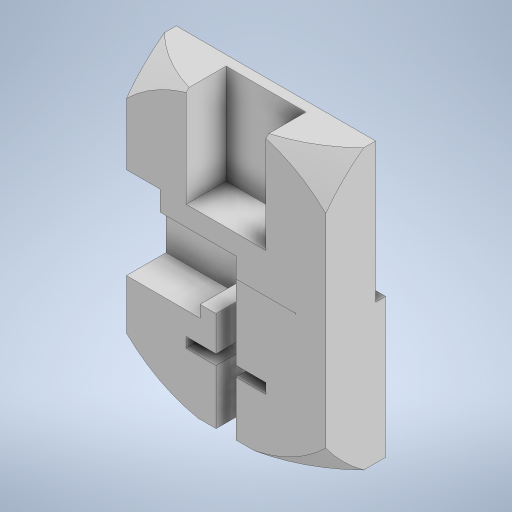
# Autodesk Inventor part: bunny head anchor
Saved by Autodesk Inventor 2024.2 (Build 282272000, 272)
## iProperties
Created: 2025-12-17
Part Number: bunny head anchor
Material: Generic
Document SubType Name: Modeling
Designer: David Toler II
Density: 1 g/cm^3
Appearance: Default
Author: David Toler II
Autodesk Inventor part; units mm, degrees
ref_plane "YZ Plane" through (0, 0, 0) normal (1, 0, 0) x (0, 1, 0)
ref_plane "XZ Plane" through (0, 0, 0) normal (0, 1, 0) x (-1, 0, 0)
ref_plane "XY Plane" through (0, 0, 0) normal (0, 0, 1) x (1, 0, 0)
sketch "Sketch1" plane through (0, 0, 0) normal (0, 0, 1) x (1, 0, 0)
  line L0 (31.75, -44.45) -> (-31.75, -44.45)
  line L1 (-31.75, -44.45) -> (-31.75, 44.45)
  line L2 (-31.75, 44.45) -> (31.75, 44.45)
  line L3 (31.75, 44.45) -> (31.75, -44.45)
  line L4 (31.75, -44.45) -> (-31.75, 44.45) construction
  line L5 (-31.75, -44.45) -> (31.75, 44.45) construction
  line L6 (-31.75, 0) -> (31.75, 0)
  line L7 (-31.75, 44.45) -> (31.75, 0)
  line L8 (-31.75, 0) -> (31.75, 44.45)
  circle A0 centre (0, 22.225) radius 11.43
  point P0 (0, 0)
  dimension "d0" = 63.5
  dimension "d1" = 44.45
  dimension "d2" = 22.86
  constraints: 18 end point, 5 midpoint, 2 parallel, 1 centre point, 1 horizontal, 1 perpendicular
  measures "d0" distance between parallel lines of L3 L1
  measures "d1" distance from line of point (0, 0) L2
  measures "d2" diameter of A0
extrude "Extrusion1" add sketch "Sketch1" along normal blind 3.175 contours L0 L1 L6 L3 | A0 L8 L7 | L7 L8 A0 | A0 L7 L8 | L8 L7 A0
sketch "Sketch2" plane through (0, 0, 3.175) normal (0, 0, 1) x (1, 0, 0)
  line L0 (31.75, -44.45) -> (31.75, 0) projected
  line L1 (31.75, 0) -> (-31.75, 0) projected
  line L2 (-31.75, 0) -> (-31.75, -44.45) projected
  line L3 (-31.75, -44.45) -> (31.75, -44.45) projected
  line L4 (-31.75, 44.45) -> (31.75, 44.45)
  line L5 (31.75, 44.45) -> (31.75, -44.45)
  line L6 (31.75, -44.45) -> (-31.75, -44.45)
  line L7 (-31.75, -44.45) -> (-31.75, 44.45)
  line L8 (-31.75, 44.45) -> (31.75, -44.45) construction
  line L9 (31.75, 44.45) -> (-31.75, -44.45) construction
  point P0 (0, 0)
  constraints: 12 end point, 2 midpoint, 2 parallel, 1 horizontal, 1 perpendicular
extrude "Extrusion2" add sketch "Sketch2" along normal blind 3.175
sketch "Sketch3" plane through (0, 0, 6.35) normal (0, 0, 1) x (1, 0, 0)
  circle A0 centre (0, -0.4493) radius 54.991
  line L0 (0, -0.4493) -> (0, 0)
  line L1 (31.75, -44.45) -> (31.75, 44.45) projected
  line L2 (31.75, 44.45) -> (-31.75, 44.45) projected
  line L3 (-31.75, 44.45) -> (-31.75, -44.45) projected
  line L4 (-31.75, -44.45) -> (31.75, -44.45) projected
  line L5 (-31.75, -44.45) -> (31.75, -44.45) projected
  line L6 (0, 44.45) -> (0, -44.45)
  line L7 (31.75, 0) -> (-31.75, 0) projected
  line L8 (-31.75, 0) -> (31.75, 0)
  line L9 (12.7, 12.7) -> (-12.7, 12.7)
  line L10 (-12.7, 12.7) -> (-12.7, 44.45)
  line L11 (-12.7, 44.45) -> (12.7, 44.45)
  line L12 (12.7, 44.45) -> (12.7, 12.7)
  line L13 (12.7, 12.7) -> (-12.7, 44.45) construction
  line L14 (-12.7, 12.7) -> (12.7, 44.45) construction
  line L15 (-33.655, 6.35) -> (-8.255, 6.35)
  line L16 (-8.255, 6.35) -> (-8.255, -16.51)
  line L17 (-8.255, -16.51) -> (-33.655, -16.51)
  line L18 (-33.655, -16.51) -> (-33.655, 6.35)
  line L19 (-8.255, 6.35) -> (31.75, 6.35)
  line L20 (-8.255, -12.7) -> (-3.175, -12.7)
  line L21 (-3.175, -12.7) -> (-3.175, -44.45)
  line L22 (-20.955, 6.35) -> (-20.955, 12.7)
  line L23 (-20.955, 12.7) -> (-31.75, 12.7)
  line L24 (3.175, 6.35) -> (3.175, -44.45)
  point P0 (0, -55.4403)
  point P1 (0, 28.575)
  point P2 (3.175, -44.45)
  point P3 (-3.175, -44.45)
  point P4 (-31.75, -16.51)
  dimension "d8" = 109.982
  dimension "d9" = 25.4
  dimension "d10" = 31.75
  dimension "d11" = 25.4
  dimension "d12" = 8.255
  dimension "d13" = 6.35
  dimension "d14" = 22.86
  dimension "d15" = 5.08
  dimension "d16" = 19.05
  dimension "d17" = 6.35
  constraints: 38 end point, 9 point on line, 6 perpendicular, 5 midpoint, 4 horizontal, 4 parallel, 2 point on circle, 2 vertical, 1 centre point
  measures "d8" diameter of A0
  measures "d9" distance between parallel lines of L12 L10
  measures "d10" distance of L9.end L10.end
  measures "d11" distance between parallel lines of L16 L18
  measures "d12" distance between parallel lines of L6 L16
  measures "d13" distance between parallel lines of L7 L15
  measures "d14" distance between parallel lines of L15 L17
  measures "d15" distance between parallel lines of L21 L16
  measures "d16" distance between parallel lines of L19 L20
  measures "d17" distance between parallel lines of L24 L21
extrude "Extrusion3" add sketch "Sketch3" along normal blind 12.7 contours L1 L19 L6 L9 L12 L2 | L2 L10 L9 L6 L19 L15 L22 L23 L3 | L1 L7 L24 L19 | L1 L4 L24 L7 | L17 L16 L20 L21 L4 L3
sketch "Sketch4" plane through (0, 0, 19.05) normal (0, 0, 1) x (1, 0, 0)
  line L0 (-20.955, 12.7) -> (-20.955, 6.35) projected
  line L1 (-20.955, 6.35) -> (3.175, 6.35) projected
  line L2 (3.175, 6.35) -> (3.175, -44.45) projected
  line L3 (3.175, -44.45) -> (31.75, -44.45) projected
  line L4 (31.75, -44.45) -> (31.75, 44.45) projected
  line L5 (31.75, 44.45) -> (12.7, 44.45) projected
  line L6 (12.7, 44.45) -> (12.7, 12.7) projected
  line L7 (12.7, 12.7) -> (-12.7, 12.7) projected
  line L8 (-12.7, 12.7) -> (-12.7, 44.45) projected
  line L9 (-12.7, 44.45) -> (-31.75, 44.45) projected
  line L10 (-31.75, 44.45) -> (-31.75, 12.7) projected
  line L11 (-31.75, 12.7) -> (-20.955, 12.7) projected
  line L12 (-3.175, -12.7) -> (-8.255, -12.7) projected
  line L13 (-8.255, -12.7) -> (-8.255, -16.51) projected
  line L14 (-8.255, -16.51) -> (-31.75, -16.51) projected
  line L15 (-31.75, -16.51) -> (-31.75, -44.45) projected
  line L16 (-31.75, -44.45) -> (-3.175, -44.45) projected
  line L17 (-3.175, -44.45) -> (-3.175, -12.7) projected
  line L18 (3.175, -44.45) -> (3.175, 6.35) projected
  line L19 (3.175, 6.35) -> (-20.955, 6.35) projected
  line L20 (-20.955, 6.35) -> (-20.955, 12.7) projected
  line L21 (-20.955, 12.7) -> (-31.75, 12.7) projected
  line L22 (-31.75, 12.7) -> (-31.75, -16.51) projected
  line L23 (-31.75, -16.51) -> (-8.255, -16.51) projected
  line L24 (-8.255, -16.51) -> (-8.255, -12.7) projected
  line L25 (-8.255, -12.7) -> (-3.175, -12.7) projected
  line L26 (-3.175, -12.7) -> (-3.175, -44.45) projected
  line L27 (-3.175, -44.45) -> (3.175, -44.45) projected
  line L28 (31.75, 0) -> (-31.75, 0) projected
  line L29 (-31.75, -25.4) -> (31.75, -25.4)
  line L30 (0, 0) -> (0, -44.45)
  line L31 (12.7, -26.9875) -> (-12.7, -26.9875)
  line L32 (-12.7, -26.9875) -> (-12.7, -23.8125)
  line L33 (-12.7, -23.8125) -> (12.7, -23.8125)
  line L34 (12.7, -23.8125) -> (12.7, -26.9875)
  line L35 (12.7, -26.9875) -> (-12.7, -23.8125) construction
  line L36 (-12.7, -26.9875) -> (12.7, -23.8125) construction
  point P0 (0, -25.4)
  dimension "d20" = 25.4
  dimension "d21" = 3.175
  dimension "d22" = 25.4
  constraints: 16 end point, 4 midpoint, 3 point on line, 2 parallel, 2 perpendicular, 1 horizontal
  measures "d20" distance between parallel lines of L29 L28
  measures "d21" distance of L31.end L32.end
  measures "d22" distance of L31.start L31.end
extrude "Extrusion4" cut sketch "Sketch4" against normal blind 9.525 contours L33 L34 L29 L2 | L2 L29 L30 L33 | L30 L29 L17 L33 | L29 L34 L31 L2 | L2 L31 L30 L29 | L32 L33 L17 L29 | L29 L17 L31 L32 | L30 L31 L17 L29
sketch "Sketch5" plane through (0, 0, 0) normal (0, 1, 0) x (-1, 0, 0)
  line L0 (-31.75, 3.175) -> (31.75, 3.175) projected
  line L1 (31.75, 3.175) -> (31.75, 19.05) projected
  line L2 (12.7, 19.05) -> (31.75, 19.05) projected
  line L3 (12.7, 6.35) -> (12.7, 19.05) projected
  line L4 (-12.7, 6.35) -> (12.7, 6.35) projected
  line L5 (-12.7, 6.35) -> (-12.7, 19.05) projected
  line L6 (-31.75, 19.05) -> (-12.7, 19.05) projected
  line L7 (-31.75, 3.175) -> (-31.75, 19.05) projected
  circle A0 centre (0, -25.4) radius 63.5
  line L8 (0, 0) -> (0, -25.4)
  circle A1 centre (0, -25.4) radius 114.3
  line L9 (0, -25.4) -> (114.3, -25.4)
  line L10 (0, -25.4) -> (0, 88.9)
  point P0 (0, 38.1)
  point P1 (63.5, -25.4)
  dimension "d25" = 28.575
  dimension "d26" = 127
  dimension "d27" = 50.8
  constraints: 6 end point, 2 centre point, 2 point on circle, 1 coincident, 1 horizontal, 1 perpendicular, 1 vertical
  measures "d25" distance from line of L8.end L0
  measures "d26" diameter of A0
  measures "d27" radial gap between concentric circles of A0 A1
revolve "Revolution1" cut sketch "Sketch5" angle 360 about axis through (0, 0, -25.4) along (0, 0, 1) picked at (44.2136, 61.1262) contours L10 A1 L9 A0
sketch "Sketch7" plane through (3.175, -44.45, 6.35) normal (-1, 0, 0) x (0, 0, 1)
  arc A0 (0.6288, 0) -> (12.7, 12.0712) centre (-31.75, 44.45) ccw projected
  line L0 (-6.35, 0) -> (0.6288, 0) projected
  line L1 (-6.35, 0) -> (-6.35, 44.45) projected
  line L2 (-6.35, 44.45) -> (-3.175, 44.45) projected
  line L3 (-3.175, 44.45) -> (-3.175, 88.9) projected
  line L4 (-3.175, 88.9) -> (0.6288, 88.9) projected
  arc A1 (12.7, 76.8288) -> (0.6288, 88.9) centre (-31.75, 44.45) ccw projected
  line L5 (12.7, 12.0712) -> (12.7, 76.8288) projected
  line L6 (0, 50.8) -> (12.7, 50.8) projected
  line L7 (12.7, 20.6375) -> (3.175, 20.6375) projected
  line L8 (12.7, 17.4625) -> (3.175, 17.4625) projected
  circle A2 centre (6.35, 44.45) radius 6.35
  circle A3 centre (4.7625, 19.05) radius 1.5875
  line L9 (3.175, 20.6375) -> (3.175, 17.4625) projected
  line L10 (12.7, 20.6375) -> (3.175, 20.6375) projected
  circle A4 centre (6.35, 44.45) radius 2.4478
  dimension "d37" = 12.7
  dimension "d38" = 3.175
  constraints: 4 tangent, 3 centre point, 1 coincident
  measures "d37" diameter of A2
  measures "d38" diameter of A3
extrude "Extrusion5" cut sketch "Sketch7" along normal mid plane 38.1 contours A3 | A2 | A4
body "Solid1"
